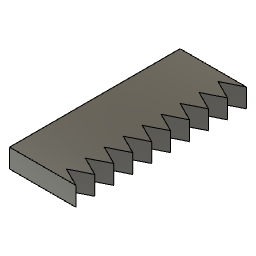
DDI_BUT_P-.5mm v1 (Autodesk Fusion 360 design; units mm, degrees)
Autodesk Fusion 360 part; units mm, degrees
sketch "Sketch1" plane through (0, 0, 0) normal (0, 0, 1) x (1, 0, 0)
  line L0 (0, 0) -> (4, 0)
  line L1 (4, 0) -> (4, 9)
  line L2 (4, 9) -> (0, 9)
  line L3 (0, 9) -> (0, 0)
  line L4 (4, 9) -> (3, 8.5)
  line L5 (3, 8.5) -> (4, 8)
  line L6 (4, 8) -> (3, 7.5)
  line L7 (3, 7.5) -> (4, 7)
  line L8 (4, 7) -> (3, 6.5)
  line L9 (3, 6.5) -> (4, 6)
  line L10 (4, 6) -> (3, 5.5)
  line L11 (3, 5.5) -> (4, 5)
  line L12 (4, 5) -> (3, 4.5)
  line L13 (3, 4.5) -> (4, 4)
  line L14 (4, 4) -> (3, 3.5)
  line L15 (3, 3.5) -> (4, 3)
  line L16 (4, 3) -> (3, 2.5)
  line L17 (3, 2.5) -> (4, 2)
  line L18 (4, 2) -> (3, 1.5)
  line L19 (3, 1.5) -> (4, 1)
  line L20 (4, 1) -> (3, 0.5)
  line L21 (3, 0.5) -> (4, 0)
  dimension "d1" = 4
  dimension "d2" = 9
  constraint horizontal L0
  constraint vertical L1
  constraint horizontal L2
  constraint vertical L3
  constraint coincident L0.start L3.end
  constraint coincident L1 L5.end
  constraint parallel L4 L6
  constraint coincident L1 L7.end
  constraint parallel L5 L7
  constraint parallel L6 L8
  constraint coincident L1 L9.end
  constraint parallel L7 L9
  constraint parallel L8 L10
  constraint coincident L1 L11.end
  constraint parallel L9 L11
  constraint parallel L10 L12
  constraint coincident L1 L13.end
  constraint parallel L11 L13
  constraint parallel L12 L14
  constraint coincident L1 L15.end
  constraint parallel L13 L15
  constraint parallel L14 L16
  constraint coincident L1 L17.end
  constraint parallel L15 L17
  constraint parallel L16 L18
  constraint coincident L1 L19.end
  constraint parallel L17 L19
  constraint parallel L18 L20
  measures "d1" distance of L0.start L0.end
  measures "d2" distance of L0.start L2.end
extrude "Extrude1" add sketch "Sketch1" along normal blind 1 contours L0 L2 L3 L4 L5 L6 L7 L8 L9 L10 L11 L12 L13 L14 L15 L16 L17 L18 L19 L20 L21
extrude "Extrude2" cut 1 faces at (0, 6, 0.3333) along direction (1, 0, 0) blind 0.5
